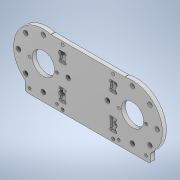
# Autodesk Inventor part: Trunk_horizontal_frame_01
Saved by Autodesk Inventor 2020.4 (Build 244396000, 396)
## iProperties
Created: 2021-09-21
Part Number: Trunk_horizontal_frame_01
Material: アルミニウム 2014-T4
Document SubType Name: Modeling
Designer: Masato Kubotera
Density: 2.8 g/cm^3
Appearance: 滑らか - 淡い灰色
Mass: 78.9795 g
Surface Area: 178.54 cm^2
Volume: 28.207 cm^3
Author: Masato Kubotera
Autodesk Inventor part; units mm, degrees
ref_plane "YZ Plane" through (0, 0, 0) normal (1, 0, 0) x (0, 1, 0)
ref_plane "XZ Plane" through (0, 0, 0) normal (0, 1, 0) x (-1, 0, 0)
ref_plane "XY Plane" through (0, 0, 0) normal (0, 0, 1) x (1, 0, 0)
sketch "スケッチ1" plane through (0, 0, 0) normal (0, 0, 1) x (1, 0, 0)
  line L0 (-62, 30.75) -> (62, 30.75)
  line L1 (62, -30.75) -> (-62, -30.75)
  line L2 (-62, 30.75) -> (62, -30.75) construction
  line L3 (62, 30.75) -> (-62, -30.75) construction
  line L4 (0, 30.75) -> (0, -30.75) construction
  circle A0 centre (-44, 2.25) radius 10.5 construction
  line L5 (-57.5, 1.25) -> (-30.5, 1.25) construction
  line L6 (-30.5, 1.25) -> (-30.5, -25.75) construction
  line L7 (-30.5, -25.75) -> (-57.5, -25.75) construction
  line L8 (-57.5, -25.75) -> (-57.5, 1.25) construction
  line L9 (-44, 1.25) -> (-44, -25.75) construction
  line L10 (-57.5, -12.25) -> (-30.5, -12.25) construction
  circle A1 centre (-57.5, 1.25) radius 1.35
  circle A2 centre (-57.5, -25.75) radius 1.35
  circle A3 centre (-30.5, 1.25) radius 1.35
  circle A4 centre (-30.5, -25.75) radius 1.35
  line L11 (-27.5, 21.75) -> (-22.5, 21.75) construction
  line L12 (-22.5, 21.75) -> (-22.5, 11.75) construction
  line L13 (-22.5, 11.75) -> (-27.5, 11.75) construction
  line L14 (-27.5, 11.75) -> (-27.5, 21.75) construction
  line L15 (-27.5, 21.75) -> (-22.5, 11.75) construction
  line L16 (-22.5, 21.75) -> (-27.5, 11.75) construction
  line L17 (-27.51, 21.76) -> (-22.49, 21.76)
  line L18 (-22.49, 21.76) -> (-22.49, 11.74)
  line L19 (-22.49, 11.74) -> (-27.51, 11.74)
  line L20 (-27.51, 11.74) -> (-27.51, 21.76)
  line L21 (-27.51, 21.76) -> (-22.49, 11.74) construction
  line L22 (-22.49, 21.76) -> (-27.51, 11.74) construction
  line L23 (-27.51, 16.75) -> (-22.49, 16.75) construction
  line L24 (-25, 21.76) -> (-25, 11.74) construction
  arc A5 (-27.51, 21.76) -> (-27.51, 19.66) centre (-27.51, 20.71) ccw
  arc A6 (-22.49, 19.66) -> (-22.49, 21.76) centre (-22.49, 20.71) ccw
  arc A7 (-27.51, 13.84) -> (-27.51, 11.74) centre (-27.51, 12.79) ccw
  arc A8 (-22.49, 11.74) -> (-22.49, 13.84) centre (-22.49, 12.79) ccw
  circle A9 centre (-25, 27.75) radius 1.55
  line L25 (-27.5, -9.25) -> (-22.5, -9.25) construction
  line L26 (-22.5, -9.25) -> (-22.5, -21.75) construction
  line L27 (-22.5, -21.75) -> (-27.5, -21.75) construction
  line L28 (-27.5, -21.75) -> (-27.5, -9.25) construction
  line L29 (-27.5, -9.25) -> (-22.5, -21.75) construction
  line L30 (-22.5, -9.25) -> (-27.5, -21.75) construction
  line L31 (-27.51, -9.24) -> (-22.49, -9.24)
  line L32 (-22.49, -9.24) -> (-22.49, -21.76)
  line L33 (-22.49, -21.76) -> (-27.51, -21.76)
  line L34 (-27.51, -21.76) -> (-27.51, -9.24)
  line L35 (-27.51, -9.24) -> (-22.49, -21.76) construction
  line L36 (-22.49, -9.24) -> (-27.51, -21.76) construction
  line L37 (-27.51, -15.5) -> (-22.49, -15.5) construction
  line L38 (-25, -9.24) -> (-25, -21.76) construction
  arc A10 (-27.51, -9.24) -> (-27.51, -11.34) centre (-27.51, -10.29) ccw
  arc A11 (-22.49, -11.34) -> (-22.49, -9.24) centre (-22.49, -10.29) ccw
  arc A12 (-22.49, -21.76) -> (-22.49, -19.66) centre (-22.49, -20.71) ccw
  arc A13 (-27.51, -19.66) -> (-27.51, -21.76) centre (-27.51, -20.71) ccw
  circle A14 centre (-25, -27.75) radius 1.55
  circle A15 centre (-44, 2.25) radius 11
  line L39 (62, 2.25) -> (-62, 2.25) construction
  line L40 (-60, 14.25) -> (-28, 14.25) construction
  line L41 (-28, 14.25) -> (-28, -28.75) construction
  line L42 (-28, -28.75) -> (-60, -28.75) construction
  line L43 (-60, -28.75) -> (-60, 14.25) construction
  line L44 (-60, 14.25) -> (-28, -28.75) construction
  line L45 (-28, 14.25) -> (-60, -28.75) construction
  line L46 (-62, 30.75) -> (-62, -30.75) construction
  line L47 (62, 30.75) -> (62, -30.75) construction
  circle A16 centre (-44, 2.25) radius 12.5 construction
  circle A17 centre (-44, 2.25) radius 20.5 construction
  circle A18 centre (-44, 2.25) radius 28.5 construction
  circle A19 centre (-44, 2.25) radius 29.5 construction
  circle A20 centre (-44, 26.75) radius 2.2
  circle A21 centre (-61.3241, 19.5741) radius 2.2
  circle A22 centre (-68.5, 2.25) radius 2.2
  circle A23 centre (-61.3241, -15.0741) radius 2.2
  circle A24 centre (-44, -22.25) radius 2.2
  circle A25 centre (-26.6759, -15.0741) radius 2.2
  circle A26 centre (-19.5, 2.25) radius 2.2
  circle A27 centre (-26.6759, 19.5741) radius 2.2
  arc A28 (-36.3842, 30.75) -> (-62, -21.122) centre (-44, 2.25) ccw
  line L48 (-62, -21.122) -> (-62, -30.75)
  circle A29 centre (57.5, 1.25) radius 1.35
  circle A30 centre (57.5, -25.75) radius 1.35
  circle A31 centre (30.5, 1.25) radius 1.35
  circle A32 centre (30.5, -25.75) radius 1.35
  line L49 (27.51, 21.76) -> (22.49, 21.76)
  line L50 (22.49, 21.76) -> (22.49, 11.74)
  line L51 (22.49, 11.74) -> (27.51, 11.74)
  line L52 (27.51, 11.74) -> (27.51, 21.76)
  arc A33 (27.51, 19.66) -> (27.51, 21.76) centre (27.51, 20.71) ccw
  arc A34 (22.49, 21.76) -> (22.49, 19.66) centre (22.49, 20.71) ccw
  arc A35 (22.49, 13.84) -> (22.49, 11.74) centre (22.49, 12.79) ccw
  arc A36 (27.51, 11.74) -> (27.51, 13.84) centre (27.51, 12.79) ccw
  circle A37 centre (25, 27.75) radius 1.55
  arc A38 (27.51, -21.76) -> (27.51, -19.66) centre (27.51, -20.71) ccw
  line L53 (22.49, -21.76) -> (27.51, -21.76)
  arc A39 (22.49, -19.66) -> (22.49, -21.76) centre (22.49, -20.71) ccw
  line L54 (27.51, -21.76) -> (27.51, -9.24)
  line L55 (22.49, -9.24) -> (22.49, -21.76)
  circle A40 centre (25, -27.75) radius 1.55
  arc A41 (22.49, -9.24) -> (22.49, -11.34) centre (22.49, -10.29) ccw
  line L56 (27.51, -9.24) -> (22.49, -9.24)
  arc A42 (27.51, -11.34) -> (27.51, -9.24) centre (27.51, -10.29) ccw
  circle A43 centre (44, 2.25) radius 11
  circle A44 centre (44, 26.75) radius 2.2
  circle A45 centre (61.3241, 19.5741) radius 2.2
  circle A46 centre (68.5, 2.25) radius 2.2
  circle A47 centre (61.3241, -15.0741) radius 2.2
  circle A48 centre (44, -22.25) radius 2.2
  circle A49 centre (26.6759, -15.0741) radius 2.2
  circle A50 centre (19.5, 2.25) radius 2.2
  circle A51 centre (26.6759, 19.5741) radius 2.2
  line L57 (62, -21.122) -> (62, -30.75)
  arc A52 (62, -21.122) -> (36.3842, 30.75) centre (44, 2.25) ccw
  line L58 (-68.5, 2.25) -> (-73.5, 2.25) construction
  circle A53 centre (-26.6759, 19.5741) radius 7.2 construction
  circle A54 centre (-19.5, 2.25) radius 7.2 construction
  circle A55 centre (-26.6759, -15.0741) radius 7.2 construction
  circle A56 centre (-44, 2.25) radius 24.5 construction
  circle A57 centre (-30.5, -25.75) radius 2.4
  point P0 (0, 0)
  point P1 (-25, 16.75)
  point P2 (-25, -15.5)
  point P3 (-22.49, 19.66)
  point P4 (-22.49, 13.84)
  point P5 (-27.51, 13.84)
  point P6 (-44, -7.25)
  point P7 (51.6158, 30.75)
  point P8 (-27.51, -17.1099)
  point P9 (-27.51, -13.0384)
  point P10 (27.51, -13.0384)
  point P11 (27.51, -17.1099)
  point P12 (27.51, -19.66)
  point P13 (22.49, 19.66)
  point P14 (28.56, 20.7099)
  point P15 (27.51, 17.5384)
  point P16 (-27.51, 17.5384)
  point P17 (-28.56, 20.7099)
  point P18 (-51.6158, 30.75)
  point P19 (-26.4271, 21.76)
  point P20 (-26.9247, 21.76)
  point P21 (-27.51, 21.6099)
  point P22 (27.51, 21.6099)
  point P23 (26.9247, 21.76)
  point P24 (26.4271, 21.76)
  dimension "d100" = 5
  dimension "d3" = 21
  dimension "d4" = 27
  dimension "d5" = 2.7
  dimension "d7" = 27
  dimension "d8" = 5
  dimension "d9" = 10
  dimension "d10" = 0.01
  dimension "d11" = 0.01
  dimension "d12" = 1.05
  dimension "d13" = 3.1
  dimension "d15" = 12.5
  dimension "d16" = 0.01
  dimension "d17" = 0.01
  dimension "d18" = 1.05
  dimension "d19" = 3.1
  dimension "d20" = 6
  dimension "d21" = 6
  dimension "d24" = 3
  dimension "d25" = 3
  dimension "d29" = 0.5
  dimension "d33" = 10.5
  dimension "d34" = 10.5
  dimension "d45" = 32
  dimension "d46" = 43
  dimension "d47" = 9.5
  dimension "d71" = 44
  dimension "d73" = 1
  dimension "d74" = 16.5
  dimension "d78" = 28.5
  dimension "d79" = 33
  dimension "d80" = 25
  dimension "d81" = 41
  dimension "d82" = 8
  dimension "d84" = 4.4
  dimension "d85" = 24.5
  dimension "d88" = 360
  dimension "d90" = 2
  dimension "d91" = 2
  dimension "d93" = 4
  dimension "d94" = 5
  dimension "d95" = 5
  dimension "d96" = 5
  dimension "d97" = 5
  dimension "d101" = 4.8
  constraints: 118 end point, 56 centre point, 56 symmetric about line, 37 point on circle, 26 midpoint, 19 point on line, 14 parallel, 12 coincident, 8 horizontal, 8 perpendicular, 2 collinear, 2 vertical, 1 vertical alignment, 55 other
  measures "d3" diameter of A0
  measures "d4" distance of L6.end L7.end
  measures "d5" diameter of A1
  measures "d7" distance of L6.end L5.end
  measures "d8" distance of L12.end L13.end
  measures "d9" distance of L11.end L12.end
  measures "d10" distance between parallel lines of L17 L11
  measures "d11" distance between parallel lines of L18 L12
  measures "d12" radius of A5
  measures "d13" diameter of A9
  measures "d15" distance of L30.start L27.start
  measures "d16" distance between parallel lines of L31 L25
  measures "d17" distance between parallel lines of L32 L26
  measures "d18" radius of A10
  measures "d19" diameter of A14
  measures "d20" vertical distance of L11.end A9.centre
  measures "d21" vertical distance of L27.start A14.centre
  measures "d24" vertical distance of L4.start A9.centre
  measures "d25" distance from line of L1 A14.centre
  measures "d29" radial gap between concentric circles of A0 A15
  measures "d33" vertical distance of L28.end A3.centre
  measures "d34" distance from line of A3.centre L13
  measures "d45" distance of L41.end L42.end
  measures "d46" distance of L40.end L41.end
  measures "d47" distance of point (-44, -7.25) A15.centre
  measures "d71" horizontal distance of point (0, 0) A0.centre
  measures "d73" distance of L9.start A15.centre
  measures "d74" horizontal distance of L11.start A0.centre
  measures "d78" distance from line of L39.end L0
  measures "d79" distance from line of L1 L39.end
  measures "d80" diameter of A16
  measures "d81" diameter of A17
  measures "d82" radial gap between concentric circles of A18 A17
  measures "d84" diameter of A20
  measures "d85" distance of A0.centre A20.centre
  measures "d90" horizontal distance of L1.end L42.end
  measures "d91" horizontal distance of L42.end L1.end
  measures "d93" distance from line of A20.centre L0
  measures "d94" distance of L58.start L58.end
  measures "d95" radial gap between concentric circles of A53 A27
  measures "d96" radial gap between concentric circles of A54 A26
  measures "d97" radial gap between concentric circles of A25 A55
  measures "d101" diameter of A57
extrude "押し出し1" add sketch "スケッチ1" along normal blind 4 contours L0 A52 L57 L1 L48 A28 | L0 A28 | A52 L0 | A57
fillet "フィレット1" radius 2 6 edges at (-62, -21.122, 2) (-62, -30.75, 2) (62, -21.122, 2) (62, -30.75, 2) (-36.3842, 30.75, 2) (36.3842, 30.75, 2)
extrude "押し出し2" add sketch "スケッチ1" along normal blind 2.1 contours L17 L18 L19 L20 A27 | A6 L18 | L20 A7 | A8 L18 | L31 L32 L33 L34 A25 | L34 A10 | A11 L32 | A12 L32 | L34 A13 | A51 L52 L51 L50 L49 | L50 A34 | A36 L52 | L50 A35 | L54 A38 | L53 L55 L56 L54 A49 | A39 L55 | A41 L55 | L54 A42
equation "\"d11\" = d10"
equation "\"d16\" = d10"
equation "\"d17\" = d16"
equation "\"d18\" = d12"
